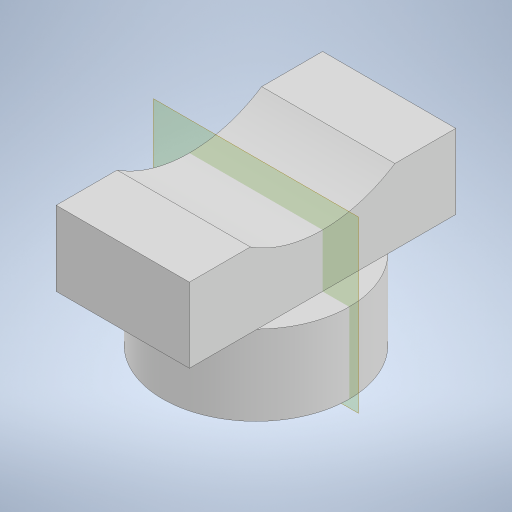
# Autodesk Inventor part: lfdbkrf
Saved by Autodesk Inventor 2023.1 (Build 271208000, 208)
## iProperties
Created: 2026-02-20
Part Number: lfdbkrf
Material: Типовые
Document SubType Name: Modeling
Designer: DELL
Density: 1 g/cm^3
Appearance: По умолчанию
Author: DELL
Autodesk Inventor part; units mm, degrees
ref_plane "YZ Plane" through (0, 0, 0) normal (1, 0, 0) x (0, 1, 0)
ref_plane "XZ Plane" through (0, 0, 0) normal (0, 1, 0) x (-1, 0, 0)
ref_plane "XY Plane" through (0, 0, 0) normal (0, 0, 1) x (1, 0, 0)
sketch "Эскиз2" plane through (0, 0, 0) normal (0, 1, 0) x (-1, 0, 0)
  circle A0 centre (0, 0) radius 2.1
  circle A1 centre (0, 0) radius 3.5
  dimension "d4" = 4.2
  dimension "d5" = 7
  constraints: 2 centre point, 2 coincident
  measures "d4" diameter of A0
  measures "d5" diameter of A1
extrude "Выдавливание2" add sketch "Эскиз2" along normal blind 3
sketch "Эскиз3" plane through (0, 3, 0) normal (0, 1, 0) x (1, 0, 0)
  line L0 (2.5, -4) -> (-2.5, -4)
  line L1 (-2.5, -4) -> (-2.5, 4)
  line L2 (-2.5, 4) -> (2.5, 4)
  line L3 (2.5, 4) -> (2.5, -4)
  circle A0 centre (0, 0) radius 2.1 projected
  line L4 (2.5, -4) -> (-2.5, 4) construction
  line L5 (-2.5, -4) -> (2.5, 4) construction
  dimension "d8" = 5
  dimension "d9" = 8
  constraints: 12 end point, 2 midpoint, 2 parallel, 1 horizontal, 1 perpendicular
  measures "d8" distance of L1.end L2.end
  measures "d9" distance of L0.end L1.end
extrude "Выдавливание3" add sketch "Эскиз3" along normal blind 2 contours L0 L1 L2 L3 | A0
sketch "Эскиз4" plane through (-2.5, 3, 4) normal (0, 0, 1) x (1, 0, 0)
  line L0 (0, 0) -> (5, 0) projected
  line L1 (0, 0) -> (5, 0)
  line L2 (5, 0) -> (5, 4)
  line L3 (5, 4) -> (0, 4)
  line L4 (0, 4) -> (0, 0)
  point P0 (2.5, -3)
  dimension "d12" = 5
  dimension "d13" = 4
  constraints: 8 end point, 2 parallel, 1 horizontal, 1 perpendicular
  measures "d12" distance of L3.end L2.end
  measures "d13" distance of L2.end L1.end
extrude "Выдавливание4" add sketch "Эскиз4" along normal blind 1
fillet "Сопряжение1" radius 5 1 edges at (0, 5, 4)
mirror "Зеркальное отражение1" about plane through (0, 0, 0) normal (0, 0, 1) of "Сопряжение1", "Выдавливание4"
sketch "Эскиз5" plane through (-2.5, 7, 5) normal (0, 1, 0) x (1, 0, 0)
  line L0 (5, 2.5505) -> (5, 0) projected
  line L1 (5, 0) -> (0, 0)
  line L2 (0, 0) -> (0, 10)
  line L3 (0, 10) -> (5, 10)
  line L4 (5, 10) -> (5, 0)
  point P0 (2.5, 5)
  point P1 (5, 5)
  constraints: 8 end point, 2 parallel, 1 horizontal, 1 perpendicular
extrude "Выдавливание5" cut sketch "Эскиз5" against normal blind 1.2
ref_plane "РабПлоскость1" through (0, 0, 0) normal (0, 0, 1) x (1, 0, 0)
